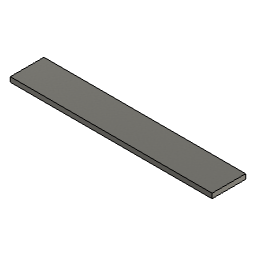
nanopositioner_assembly (Autodesk Fusion 360 archive; units mm, degrees)
design "Magnetic Tape"
part number: 2025-07-22-16-52-46-665
Autodesk Fusion 360 part; units mm, degrees
sketch "Sketch1" plane through (0, 0, 0) normal (0, 0, 1) x (1, 0, 0)
  line L0 (-30, 5) -> (30, 5)
  line L1 (30, 5) -> (30, -5)
  line L2 (30, -5) -> (-30, -5)
  line L3 (-30, -5) -> (-30, 5)
  line L4 (-30, 5) -> (30, -5) construction
  line L5 (30, 5) -> (-30, -5) construction
  dimension "d1" = 10
  dimension "d2" = 60
  constraint horizontal L0
  constraint perpendicular L0 L1
  constraint parallel L0 L2
  constraint parallel L1 L3
  constraint coincident L4 origin
  constraint coincident L5 origin
  measures "d1" distance of L0.start L2.end
  measures "d2" distance of L0.start L0.end
extrude "Extrude1" add sketch "Sketch1" along normal blind 1.43

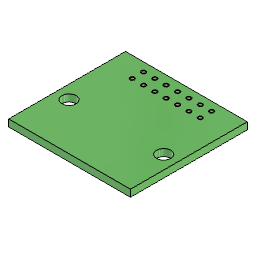
design "14 Pin Converter Board"
part number: 2025-09-17-17-01-37-446
Autodesk Fusion 360 part; units mm, degrees
sketch "Sketch1" plane through (0, 0, 0) normal (0, 0, 1) x (1, 0, 0)
  line L0 (-13.65, 13.1) -> (13.65, 13.1)
  line L1 (13.65, 13.1) -> (13.65, -13.1)
  line L2 (13.65, -13.1) -> (-13.65, -13.1)
  line L3 (-13.65, -13.1) -> (-13.65, 13.1)
  line L4 (-13.65, 13.1) -> (13.65, -13.1) construction
  line L5 (13.65, 13.1) -> (-13.65, -13.1) construction
  circle A0 centre (-10.6, -2.6) radius 1.5875
  circle A1 centre (10.6, -2.6) radius 1.5875
  dimension "d1" = 27.3
  dimension "d2" = 26.2
  dimension "d3" = 3.175
  dimension "d4" = 21.2
  dimension "d5" = 3.05
  dimension "d6" = 10.5
  constraint horizontal L0
  constraint perpendicular L0 L1
  constraint parallel L0 L2
  constraint parallel L1 L3
  constraint coincident L4 origin
  constraint coincident L5 origin
  constraint horizontal A0.centre A1.centre
  constraint equal A0 A1
  measures "d1" distance of L0.start L0.end
  measures "d2" distance of L0.start L2.end
  measures "d3" diameter of A1
  measures "d4" distance of A0.centre A1.centre
  measures "d5" distance of L3 A0.centre
  measures "d6" distance of L2 A0.centre
extrude "Extrude1" add sketch "Sketch1" along normal blind 1.5875 makes body 1
sketch "Sketch2" plane through (0, 0, 1.5875) normal (0, 0, 1) x (-1, 0, 0)
  circle A0 centre (-10.6, 2.6) radius 1.5875
  circle A1 centre (10.6, 2.6) radius 1.5875
  line L0 (13.65, 13.1) -> (-13.65, 13.1)
  line L1 (-13.65, 13.1) -> (-13.65, -13.1)
  line L2 (-13.65, -13.1) -> (13.65, -13.1)
  line L3 (13.65, -13.1) -> (13.65, 13.1)
  circle A2 centre (7.62, -11.1) radius 0.5
  circle A3 centre (5.08, -11.1) radius 0.5
  circle A4 centre (2.54, -11.1) radius 0.5
  circle A5 centre (0, -11.1) radius 0.5
  circle A6 centre (-2.54, -11.1) radius 0.5
  circle A7 centre (-5.08, -11.1) radius 0.5
  circle A8 centre (-7.62, -11.1) radius 0.5
  circle A9 centre (7.62, -8.56) radius 0.5
  circle A10 centre (5.08, -8.56) radius 0.5
  circle A11 centre (2.54, -8.56) radius 0.5
  circle A12 centre (0, -8.56) radius 0.5
  circle A13 centre (-2.54, -8.56) radius 0.5
  circle A14 centre (-5.08, -8.56) radius 0.5
  circle A15 centre (-7.62, -8.56) radius 0.5
  line L4 (13.65, -13.1) -> (-13.65, -13.1)
  dimension "d9" = 1
  dimension "d12" = -2.54
  dimension "d13" = 2.54
  dimension "d14" = 2
  constraint vertical A5.centre origin
  measures "d9" diameter of A2
  measures "d14" distance of A2.centre L4
extrude "Extrude2" cut sketch "Sketch2" against normal blind 5 contours A2 | A3 | A4 | A5 | A6 | A7 | A8 | A9 | A10 | A11 | A12 | A13 | A14 | A15 bodies 1
sketch "Sketch3" plane through (0, 0, 1.5875) normal (0, 0, 1) x (-1, 0, 0)
  circle A0 centre (0, -8.56) radius 0.5
  circle A1 centre (7.62, -8.56) radius 0.5
  circle A2 centre (0, -11.1) radius 0.5
  circle A3 centre (7.62, -11.1) radius 0.5
  circle A4 centre (-2.54, -11.1) radius 0.5
  circle A5 centre (5.08, -8.56) radius 0.5
  circle A6 centre (-5.08, -8.56) radius 0.5
  circle A7 centre (-2.54, -8.56) radius 0.5
  circle A8 centre (-7.62, -11.1) radius 0.5
  circle A9 centre (2.54, -11.1) radius 0.5
  circle A10 centre (5.08, -11.1) radius 0.5
  circle A11 centre (-5.08, -11.1) radius 0.5
  circle A12 centre (2.54, -8.56) radius 0.5
  circle A13 centre (-7.62, -8.56) radius 0.5
  circle A14 centre (-10.6, 2.6) radius 1.5875
  circle A15 centre (10.6, 2.6) radius 1.5875
  line L0 (13.65, 13.1) -> (-13.65, 13.1)
  line L1 (-13.65, 13.1) -> (-13.65, -13.1)
  line L2 (-13.65, -13.1) -> (13.65, -13.1)
  line L3 (13.65, -13.1) -> (13.65, 13.1)
  circle A16 centre (-7.62, -8.56) radius 0.35
  circle A17 centre (-5.08, -8.56) radius 0.35
  circle A18 centre (-2.54, -8.56) radius 0.35
  circle A19 centre (0, -8.56) radius 0.35
  circle A20 centre (2.54, -8.56) radius 0.35
  circle A21 centre (5.08, -8.56) radius 0.35
  circle A22 centre (7.62, -8.56) radius 0.35
  circle A23 centre (-7.62, -11.1) radius 0.35
  circle A24 centre (-5.08, -11.1) radius 0.35
  circle A25 centre (-2.54, -11.1) radius 0.35
  circle A26 centre (0, -11.1) radius 0.35
  circle A27 centre (2.54, -11.1) radius 0.35
  circle A28 centre (5.08, -11.1) radius 0.35
  circle A29 centre (7.62, -11.1) radius 0.35
  dimension "d17" = 0.7
  dimension "d20" = 2.54
  dimension "d21" = -2.54
  constraint concentric A13 A16
  measures "d17" diameter of A16
extrude "Extrude3" add sketch "Sketch3" against normal blind 3 separate body contours A16 | A17 | A18 | A19 | A20 | A21 | A22 | A23 | A24 | A25 | A26 | A27 | A28 | A29 makes body 2 at (-2.1917, 11.1348, -0.4125) makes body 3 at (-2.1917, 8.5948, -0.4125) makes body 4 at (-7.9187, 11.2825, -0.4125) makes body 5 at (4.7813, 8.7425, -0.4125) makes body 6 at (0.3483, 8.5948, -0.4125) makes body 7 at (-5.3787, 11.2825, -0.4125) makes body 8 at (2.8883, 8.5948, -0.4125) makes body 9 at (0.3483, 11.1348, -0.4125) makes body 10 at (7.3213, 8.7425, -0.4125) makes body 11 at (7.3213, 11.2825, -0.4125) makes body 12 at (-7.9187, 8.7425, -0.4125) makes body 13 at (4.7813, 11.2825, -0.4125) makes body 14 at (2.8883, 11.1348, -0.4125) makes body 15 at (-5.3787, 8.7425, -0.4125)
equation "d5 = ( d1 - d4 ) / 2"
